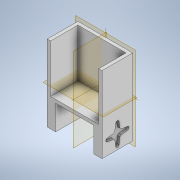
# Autodesk Inventor part: Block
Saved by Autodesk Inventor 2021 (Build 250183000, 183)
## iProperties
Created: 2022-11-29
Part Number: Block
Material: Generisch
Document SubType Name: Modeling
Designer: Elian
Density: 1 g/cm^3
Appearance: Vorgabe
Author: Elian
Autodesk Inventor part; units mm, degrees
sketch "Skizze1" plane through (0, 0, 0) normal (0, 0, 1) x (1, 0, 0)
  line L0 (-33, 46) -> (33, 46)
  line L1 (33, 46) -> (33, -46)
  line L2 (33, -46) -> (-33, -46)
  line L3 (-33, -46) -> (-33, 46)
  line L4 (0, -64.4) -> (0, 64.4) projected
  line L5 (-46.2, 0) -> (46.2, 0) projected
  point P0 (0, 0)
  dimension "d0" = 66
  dimension "d1" = 92
  constraints: 8 end point, 2 parallel, 1 horizontal, 1 perpendicular, 2 other
  measures "d0" distance of L1.end L2.end
  measures "d1" distance of L0.end L1.end
extrude "Extrusion1" add sketch "Skizze1" along normal blind 37
sketch "Skizze2" plane through (0, 0, 37) normal (0, 0, 1) x (1, 0, 0)
  line L0 (-33, -46) -> (33, -46) projected
  line L1 (-23, -46) -> (23, -46)
  line L2 (23, -46) -> (23, -16)
  line L3 (23, -16) -> (-23, -16)
  line L4 (-23, -16) -> (-23, -46)
  line L5 (0, -64.4) -> (0, 64.4) projected
  point P0 (0, 0)
  dimension "d4" = 46
  dimension "d5" = 30
  constraints: 8 end point, 2 parallel, 1 horizontal, 1 perpendicular, 1 point on line, 1 other
  measures "d4" distance of L3.end L2.end
  measures "d5" distance of L2.end L1.end
extrude "Extrusion2" cut sketch "Skizze2" against normal blind 37
sketch "Skizze3" plane through (0, 0, 37) normal (0, 0, 1) x (1, 0, 0)
  line L0 (33, 46) -> (-33, 46) projected
  line L1 (-29, 46) -> (29, 46)
  line L2 (29, 46) -> (29, -12)
  line L3 (29, -12) -> (-29, -12)
  line L4 (-29, -12) -> (-29, 46)
  line L5 (0, -64.4) -> (0, 64.4) projected
  point P0 (0, 0)
  dimension "d8" = 58
  dimension "d9" = 58
  constraints: 8 end point, 2 parallel, 1 horizontal, 1 perpendicular, 1 point on line, 1 other
  measures "d8" distance of L2.end L3.end
  measures "d9" distance of L1.end L2.end
extrude "Extrusion3" cut sketch "Skizze3" against normal blind 33
sketch "Skizze9" plane through (33, -46, 0) normal (1, 0, 0) x (0, 0, -1)
  line L0 (-18.5, 4.5) -> (-18.5, 28.5) construction
  line L1 (-16.5, 4.5) -> (-16.5, 28.5)
  line L2 (-20.5, 28.5) -> (-20.5, 4.5)
  arc A0 (-20.5, 4.5) -> (-16.5, 4.5) centre (-18.5, 4.5) ccw
  arc A1 (-16.5, 28.5) -> (-20.5, 28.5) centre (-18.5, 28.5) ccw
  line L3 (0, 0) -> (-37, 0) projected
  line L4 (0, 0) -> (0, 92) projected
  line L5 (-30.5, 16.5) -> (-6.5, 16.5) construction
  line L6 (-30.5, 14.5) -> (-6.5, 14.5)
  line L7 (-6.5, 18.5) -> (-30.5, 18.5)
  arc A2 (-30.5, 18.5) -> (-30.5, 14.5) centre (-30.5, 16.5) ccw
  arc A3 (-6.5, 14.5) -> (-6.5, 18.5) centre (-6.5, 16.5) ccw
  line L8 (-21.5851, 21.2663) -> (-20.5, 28.5)
  line L9 (-15.4149, 21.2663) -> (-16.5, 28.5)
  line L10 (-21.5851, 11.7337) -> (-20.5, 4.5)
  line L11 (-15.4149, 11.7337) -> (-16.5, 4.5)
  line L12 (-23.2663, 19.5851) -> (-30.5, 18.5)
  line L13 (-23.2663, 13.4149) -> (-30.5, 14.5)
  line L14 (-13.7337, 19.5851) -> (-6.5, 18.5)
  line L15 (-13.7337, 13.4149) -> (-6.5, 14.5)
  arc A4 (-23.2663, 19.5851) -> (-21.5851, 21.2663) centre (-23.5629, 21.5629) ccw
  arc A5 (-15.4149, 21.2663) -> (-13.7337, 19.5851) centre (-13.4371, 21.5629) ccw
  arc A6 (-13.7337, 13.4149) -> (-15.4149, 11.7337) centre (-13.4371, 11.4371) ccw
  arc A7 (-21.5851, 11.7337) -> (-23.2663, 13.4149) centre (-23.5629, 11.4371) ccw
  point P0 (0, 46)
  point P1 (-18.5, 16.5)
  point P2 (-18.5, 16.5)
  point P3 (-22, 18.5)
  point P4 (-15, 18.5)
  point P5 (-22, 14.5)
  point P6 (-15, 14.5)
  point P7 (-20.5, 20)
  point P8 (-20.5, 13)
  point P9 (-16.5, 20)
  point P10 (-16.5, 13)
  point P11 (-20.5, 4.5)
  point P12 (-16.5, 4.5)
  dimension "d59" = 4.5
  dimension "d60" = 2
  dimension "d62" = 4
  dimension "d63" = 24
  dimension "d65" = 24
  dimension "d66" = 2
  constraints: 32 end point, 17 point on circle, 16 tangent, 10 point on line, 9 symmetric about line, 8 centre point, 3 equal radius, 2 midpoint, 2 parallel, 1 perpendicular, 1 vertical, 1 other
  measures "d59" distance from line of L3 L0.start
  measures "d60" radius of A1
  measures "d62" diameter of A3
  measures "d63" distance of L7.start L7.end
  measures "d65" distance of L1.start L1.end
  measures "d66" radius of A4
extrude "Extrusion5" cut sketch "Skizze9" against normal blind 3
